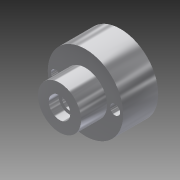
# Autodesk Inventor part: Pneumatic Connector - Bearing Hold
Saved by Autodesk Inventor 2013 (Build 170138000, 138)
## iProperties
Created: 2013-08-24
Part Number: Pneumatic Connector - Bearing Hold
Material: Generic
Document SubType Name: Modeling
Designer: grtstudent
Density: 1 g/cm^3
Author: grtstudent
Autodesk Inventor part; units mm, degrees
ref_plane "YZ Plane" through (0, 0, 0) normal (1, 0, 0) x (0, 1, 0)
ref_plane "XZ Plane" through (0, 0, 0) normal (0, 1, 0) x (-1, 0, 0)
ref_plane "XY Plane" through (0, 0, 0) normal (0, 0, 1) x (1, 0, 0)
sketch "Sketch1" plane through (0, 0, 0) normal (0, 0, 1) x (1, 0, 0)
  circle A0 centre (0, 0) radius 4.7625
  circle A1 centre (0, 0) radius 3.175
  dimension "d0" = 6.35
  dimension "d2" = 9.525
  constraints: 2 centre point, 2 coincident
  measures "d0" diameter of A1
  measures "d2" diameter of A0
extrude "Extrusion1" add sketch "Sketch1" against normal blind 1.5875
sketch "Sketch2" plane through (0, 0, -1.5875) normal (0, 0, -1) x (-1, 0, 0)
  circle A0 centre (0, 0) radius 4.7625 projected
  circle A1 centre (0, 0) radius 6.35
  dimension "d5" = 12.7
  constraints: 1 centre point, 1 coincident
  measures "d5" diameter of A1
extrude "Extrusion2" add sketch "Sketch2" along normal blind 1.5875 contours A0 | A1
sketch "Sketch3" plane through (0, 0, -3.175) normal (0, 0, -1) x (-1, 0, 0)
  circle A0 centre (0, 0) radius 6.35 projected
  circle A1 centre (0, 0) radius 3.9688
  dimension "d9" = 7.9375
  constraints: 2 coincident, 1 centre point
  measures "d9" diameter of A1
extrude "Extrusion3" add sketch "Sketch3" along normal blind 2.54
hole "Hole1" at (0, 0, -3.175) direction (0, 0, 1) diameter 4.318 depth 25.4 tip angle 118 clearance for "Flat Head Machine Screw (82)" size "#8" standard "Ansi Unified Screw Threads"
sketch "Sketch4" plane through (0, 0, -5.715) normal (0, 0, -1) x (-1, 0, 0)
  circle A0 centre (0, 0) radius 3.9687 projected
  circle A1 centre (0, 0) radius 6.35 projected
  circle A2 centre (0, 0) radius 11.1125
  dimension "d21" = 22.225
  constraints: 1 centre point, 1 coincident
  measures "d21" diameter of A2
extrude "Extrusion4" add sketch "Sketch4" along normal blind 5.969 contours A1 | A2
sketch "Sketch5" plane through (0, 0, -11.684) normal (0, 0, -1) x (-1, 0, 0)
  circle A0 centre (0, 0) radius 11.1125 projected
  circle A1 centre (0, 0) radius 6.35
  dimension "d25" = 12.7
  constraints: 1 centre point, 1 coincident
  measures "d25" diameter of A1
extrude "Extrusion5" add sketch "Sketch5" along normal blind 4.9784
sketch "Sketch9" plane through (0, 0, -5.715) normal (0, 0, 1) x (1, 0, 0)
  circle A0 centre (0, 0) radius 11.1125 projected
  circle A1 centre (0, 0) radius 6.35 projected
  line L0 (-8.7312, 0) -> (0, 0) construction
  line L1 (0, 0) -> (8.7312, 0) construction
  circle A2 centre (0, 0) radius 8.7312 construction
  dimension "d53" = 2.3813
  dimension "d54" = 2.3813
  constraints: 4 end point, 2 point on circle, 1 centre point, 1 coincident, 1 collinear, 1 horizontal
  measures "d53" radial gap between concentric circles of A1 A2
  measures "d54" radial gap between concentric circles of A0 A2
hole "Hole4" at (-8.7312, 0, -5.715) at (8.7312, 0, -5.715) direction (0, 0, -1) diameter 2.9464 end through all clearance for "Socket Head Cap Screw" size "#4" standard "Ansi Unified Screw Threads"
sketch "Sketch10" plane through (0, 0, -5.715) normal (0, 0, 1) x (1, 0, 0)
  circle A0 centre (-8.7312, 0) radius 1.4732 projected
  circle A1 centre (8.7312, 0) radius 1.4732 projected
  circle A2 centre (0, 0) radius 11.1125 projected
  circle A3 centre (0, 0) radius 6.35 projected
extrude "Extrusion6" add sketch "Sketch10" along normal blind 0.9588
sketch "Sketch11" plane through (0, 0, -1.5875) normal (0, 0, 1) x (1, 0, 0)
  circle A0 centre (0, 0) radius 6.35 projected
  circle A1 centre (0, 0) radius 3.175 projected
extrude "Extrusion7" add sketch "Sketch11" along normal blind 2.8914
sketch "Sketch12" plane through (0, 0, -4.7561) normal (0, 0, 1) x (1, 0, 0)
  circle A0 centre (0, 0) radius 6.35 projected
  circle A1 centre (8.7312, 0) radius 1.4732 projected
  circle A2 centre (-8.7312, 0) radius 1.4732 projected
  circle A3 centre (0, 0) radius 11.1125 projected
extrude "Extrusion8" cut sketch "Sketch12" against normal blind 1.5875
equation "\"d53\" = d54"
equation "\"BendRadius\" = Thickness"
equation "\"BendReliefWidth\" = Thickness"
equation "\"BendReliefDepth\" = 0.5 * Thickness"
equation "\"CornerReliefSize\" = 4 * Thickness"
equation "\"MinimumRemnant\" = 2 * Thickness"
equation "\"TransitionRadius\" = BendRadius"
equation "\"JacobiRadiusSize\" = Thickness"
equation "\"GapSize\" = Thickness"
equation "\"Thickness\" = 3.048"
body "Solid1"
